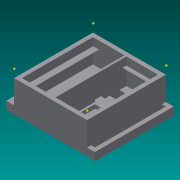
# Autodesk Inventor part: nano_enclosure_v3
Saved by Autodesk Inventor 2015 (Build 190159000, 159)
## iProperties
Created: 2015-03-02
Part Number: nano_enclosure_v3
Material: Generic
Document SubType Name: Modeling
Designer: Jeff
Density: 1 g/cm^3
Appearance: Default
Author: Jeff
Autodesk Inventor part; units mm, degrees
ref_plane "YZ Plane" through (0, 0, 0) normal (1, 0, 0) x (0, 1, 0)
ref_plane "XZ Plane" through (0, 0, 0) normal (0, 1, 0) x (-1, 0, 0)
ref_plane "XY Plane" through (0, 0, 0) normal (0, 0, 1) x (1, 0, 0)
sketch "Sketch2" plane through (0, 0, 0) normal (0, 0, 1) x (1, 0, 0)
  line L0 (0, 0) -> (46.99, 0)
  line L1 (46.99, 0) -> (46.99, 50.8)
  line L2 (46.99, 50.8) -> (0, 50.8)
  line L3 (0, 50.8) -> (0, 0)
  dimension "d0" = 50.8
  dimension "d1" = 46.99
  constraints: 8 end point, 2 parallel, 1 horizontal, 1 perpendicular
  measures "d0" distance of L0.end L1.end
  measures "d1" distance of L1.end L2.end
extrude "Extrusion1" add sketch "Sketch2" along normal blind 25.4
sketch "Sketch3" plane through (0, 0, 25.4) normal (0, 0, 1) x (1, 0, 0)
  line L0 (2.54, 2.54) -> (22.86, 2.54)
  line L1 (22.86, 2.54) -> (22.86, 48.26)
  line L2 (22.86, 48.26) -> (2.54, 48.26)
  line L3 (2.54, 48.26) -> (2.54, 2.54)
  line L4 (0, 0) -> (46.99, 0) projected
  line L5 (0, 50.8) -> (0, 0) projected
  line L6 (46.99, 50.8) -> (0, 50.8) projected
  line L7 (24.13, 2.54) -> (44.45, 2.54)
  line L8 (44.45, 2.54) -> (44.45, 48.26)
  line L9 (44.45, 48.26) -> (24.13, 48.26)
  line L10 (24.13, 48.26) -> (24.13, 2.54)
  line L11 (46.99, 0) -> (46.99, 50.8) projected
  dimension "d4" = 2.54
  dimension "d5" = 2.54
  dimension "d6" = 2.54
  dimension "d7" = 22.86
  dimension "d8" = 2.54
  dimension "d9" = 2.54
  dimension "d10" = 2.54
  dimension "d11" = 22.86
  constraints: 16 end point, 4 parallel, 2 horizontal, 2 perpendicular
  measures "d4" distance between parallel lines of L4 L0
  measures "d5" distance between parallel lines of L5 L3
  measures "d6" distance between parallel lines of L6 L2
  measures "d7" distance between parallel lines of L5 L1
  measures "d8" distance between parallel lines of L4 L7
  measures "d9" distance between parallel lines of L11 L8
  measures "d10" distance between parallel lines of L6 L9
  measures "d11" distance between parallel lines of L11 L10
extrude "Extrusion2" cut sketch "Sketch3" against normal blind 20.32 contours L3 L2 L1 L0 | L10 L9 L8 L7
sketch "Sketch4" plane through (0, 0, 0) normal (0, 0, -1) x (-1, 0, 0)
  circle A0 centre (-12.7, 17.78) radius 8.89
  line L0 (0, 50.8) -> (0, 0) projected
  line L1 (0, 0) -> (-46.99, 0) projected
  dimension "d14" = 17.78
  dimension "d17" = 12.7
  dimension "d18" = 17.78
  constraints: 1 centre point
  measures "d14" diameter of A0
  measures "d17" distance from line of L0 A0.centre
  measures "d18" distance from line of L1 A0.centre
extrude "Extrusion3" cut sketch "Sketch4" against normal blind 3.175
sketch "Sketch5" plane through (0, 0, 0) normal (0, 0, -1) x (-1, 0, 0)
  point P0 (0, 0)
sketch "Sketch6" plane through (12.7, 17.78, 3.175) normal (0, 0, -1) x (-1, 0, 0)
  circle A0 centre (0, 0) radius 8.89 projected
  line L0 (0, 0) -> (-5.08, 0)
  line L1 (-5.08, 0) -> (-5.08, 12.7)
  line L2 (-5.08, 12.7) -> (0, 12.7)
  line L3 (0, 12.7) -> (0, 0)
  line L4 (0, 0) -> (5.08, 0)
  line L5 (5.08, 0) -> (5.08, 12.7)
  line L6 (5.08, 12.7) -> (0, 12.7)
  line L7 (0, 12.7) -> (0, 0)
  point P0 (12.7, -17.78)
  dimension "d21" = 12.7
  dimension "d22" = 5.08
  dimension "d23" = 5.08
  constraints: 16 end point, 4 parallel, 2 horizontal, 2 perpendicular, 1 point on line
  measures "d21" distance between parallel lines of L4 L6
  measures "d22" distance of L0.start L0.end
  measures "d23" distance between parallel lines of L3 L5
extrude "Extrusion4" cut sketch "Sketch6" along normal blind 5.08 contours L5 L4 L3 A0 | A0 L3 L6 L5 | L1 L2 L3 A0 | A0 L3 L0 L1
sketch "Sketch7" plane through (0, 0, 3.175) normal (0, 0, -1) x (-1, 0, 0)
  point P0 (0, 0)
sketch "Sketch8" plane through (0, 0, 3.175) normal (0, 0, -1) x (-1, 0, 0)
  line L0 (-7.62, 25.0756) -> (-7.62, 30.48) projected
  line L1 (-17.78, 30.48) -> (-7.62, 30.48)
  line L2 (-7.62, 30.48) -> (-7.62, 26.67)
  line L3 (-7.62, 26.67) -> (-17.78, 26.67)
  line L4 (-17.78, 26.67) -> (-17.78, 30.48)
  point P0 (0, 0)
  dimension "d26" = 3.81
  constraints: 8 end point, 2 parallel, 1 horizontal, 1 perpendicular, 1 point on line
  measures "d26" distance between parallel lines of L1 L3
extrude "Extrusion5" cut sketch "Sketch8" against normal blind 2.54
sketch "Sketch14" plane through (44.45, 2.54, 25.4) normal (-1, 0, 0) x (0, 0, 1)
  line L0 (0, 0) -> (-20.32, 0) projected
  line L1 (0, 45.72) -> (-20.32, 45.72) projected
  line L2 (-10.16, 45.72) -> (-10.16, 43.18)
  line L3 (-10.16, 43.18) -> (-12.7, 45.72)
  line L4 (-10.16, 0) -> (-10.16, 2.54)
  line L5 (-10.16, 2.54) -> (-12.7, 0)
  point P0 (-25.4, -2.54)
  dimension "d52" = 45
  dimension "d53" = 2.54
  dimension "d54" = 2.54
  dimension "d55" = 45
  dimension "d56" = 7.62
  dimension "d57" = 7.62
  constraints: 8 end point, 2 midpoint, 2 point on line, 1 perpendicular, 1 vertical
  measures "d52" angle of L3 L2
  measures "d53" distance of L2.start L2.end
  measures "d54" distance of L4.start L4.end
  measures "d55" angle of L5 L4
  measures "d56" distance of L0.end L5.end
  measures "d57" distance of L1.end L3.end
extrude "Extrusion11" add sketch "Sketch14" along normal blind 20.32
sketch "Sketch16" plane through (2.54, 2.54, 25.4) normal (0, 1, 0) x (1, 0, 0)
  line L0 (0, 10.16) -> (3.81, 10.16)
  line L1 (3.81, 10.16) -> (0, 13.97)
  line L2 (0, 0) -> (0, 20.32) projected
  line L3 (20.32, 0) -> (20.32, 20.32)
  line L4 (20.32, 13.97) -> (16.51, 10.16)
  line L5 (16.51, 10.16) -> (20.32, 10.16)
  line L6 (20.32, 20.32) -> (0, 20.32) projected
  point P0 (-2.54, 25.4)
  dimension "d60" = 45
  dimension "d61" = 3.81
  dimension "d62" = 3.81
  dimension "d64" = 45
  dimension "d144" = 10.16
  dimension "d145" = 10.16
  constraints: 10 end point, 2 midpoint, 2 point on line, 1 horizontal, 1 parallel
  measures "d60" angle of L4 L5
  measures "d61" distance of L4.end L5.end
  measures "d62" distance of L0.start L0.end
  measures "d64" angle of L1 L0
  measures "d144" distance between parallel lines of L6 L5
  measures "d145" distance between parallel lines of L6 L0
extrude "Extrusion12" add sketch "Sketch16" along normal blind 45.72
sketch "Sketch17" plane through (0, 0, 0) normal (-1, 0, 0) x (0, 0, 1)
  line L0 (0, 50.8) -> (25.4, 50.8) projected
  line L1 (0, 0) -> (5.08, 0)
  line L2 (5.08, 0) -> (5.08, 50.8)
  line L3 (5.08, 50.8) -> (0, 50.8)
  line L4 (0, 50.8) -> (0, 0)
  dimension "d68" = 5.08
  constraints: 8 end point, 2 parallel, 1 horizontal, 1 perpendicular, 1 point on line
  measures "d68" distance between parallel lines of L4 L2
extrude "Extrusion13" add sketch "Sketch17" along normal blind 5.08
sketch "Sketch18" plane through (0, 0, 5.08) normal (0, 0, 1) x (1, 0, 0)
  line L0 (0, 50.8) -> (0, 0) projected
  line L1 (0, 2.54) -> (-2.54, 2.54)
  line L2 (-2.54, 2.54) -> (-2.54, 48.26)
  line L3 (-2.54, 48.26) -> (0, 48.26)
  line L4 (0, 48.26) -> (0, 2.54)
  line L5 (0, 50.8) -> (-5.08, 50.8) projected
  line L6 (0, 0) -> (-5.08, 0) projected
  dimension "d71" = 2.54
  dimension "d72" = 2.54
  dimension "d73" = 2.54
  constraints: 8 end point, 2 parallel, 1 horizontal, 1 perpendicular, 1 point on line
  measures "d71" distance of L2.end L3.end
  measures "d72" distance between parallel lines of L5 L3
  measures "d73" distance between parallel lines of L6 L1
extrude "Extrusion14" cut sketch "Sketch18" against normal blind 5.08
sketch "Sketch19" plane through (46.99, 0, 0) normal (1, 0, 0) x (0, 0, -1)
  line L0 (0, 50.8) -> (-25.4, 50.8) projected
  line L1 (0, 0) -> (-5.08, 0)
  line L2 (-5.08, 0) -> (-5.08, 50.8)
  line L3 (-5.08, 50.8) -> (0, 50.8)
  line L4 (0, 50.8) -> (0, 0)
  dimension "d76" = 5.08
  constraints: 8 end point, 2 parallel, 1 horizontal, 1 perpendicular, 1 point on line
  measures "d76" distance between parallel lines of L4 L2
extrude "Extrusion15" add sketch "Sketch19" along normal blind 5.08
sketch "Sketch21" plane through (46.99, 0, 5.08) normal (0, 0, 1) x (1, 0, 0)
  line L0 (0, 0) -> (0, 50.8) projected
  line L1 (0, 2.54) -> (2.54, 2.54)
  line L2 (2.54, 2.54) -> (2.54, 48.26)
  line L3 (2.54, 48.26) -> (0, 48.26)
  line L4 (0, 48.26) -> (0, 2.54)
  line L5 (0, 50.8) -> (5.08, 50.8) projected
  line L6 (0, 0) -> (5.08, 0) projected
  line L7 (5.08, 50.8) -> (5.08, 0) projected
  point P0 (-46.99, 0)
  dimension "d79" = 2.54
  dimension "d81" = 2.54
  dimension "d82" = 2.54
  constraints: 8 end point, 2 parallel, 1 horizontal, 1 perpendicular, 1 point on line
  measures "d79" distance between parallel lines of L5 L3
  measures "d81" distance between parallel lines of L6 L1
  measures "d82" distance between parallel lines of L7 L2
extrude "Extrusion16" cut sketch "Sketch21" against normal blind 5.08 contours L0 L3 L2 L1
sketch "Sketch23" plane through (0, 0, 5.08) normal (0, 0, 1) x (1, 0, 0)
  line L0 (24.13, 2.54) -> (24.13, 48.26) projected
  line L1 (24.13, 33.02) -> (44.45, 33.02)
  line L2 (44.45, 33.02) -> (44.45, 48.26)
  line L3 (44.45, 48.26) -> (24.13, 48.26)
  line L4 (24.13, 48.26) -> (24.13, 33.02)
  line L5 (24.13, 37.465) -> (31.75, 37.465)
  line L6 (31.75, 37.465) -> (31.75, 43.815)
  line L7 (31.75, 43.815) -> (24.13, 43.815)
  line L8 (24.13, 43.815) -> (24.13, 37.465)
  line L9 (44.45, 48.26) -> (39.37, 48.26)
  line L10 (39.37, 48.26) -> (39.37, 33.02)
  line L11 (39.37, 33.02) -> (44.45, 33.02)
  line L12 (44.45, 33.02) -> (44.45, 48.26)
  point P0 (0, 0)
  dimension "d91" = 15.24
  dimension "d92" = 6.35
  dimension "d93" = 7.62
  dimension "d94" = 4.445
  dimension "d95" = 4.445
  dimension "d96" = 5.08
  constraints: 24 end point, 6 parallel, 3 horizontal, 3 perpendicular, 3 point on line, 1 coincident
  measures "d91" distance between parallel lines of L3 L1
  measures "d92" distance between parallel lines of L7 L5
  measures "d93" distance between parallel lines of L0 L6
  measures "d94" distance between parallel lines of L1 L5
  measures "d95" distance between parallel lines of L3 L7
  measures "d96" distance between parallel lines of L2 L10
extrude "Extrusion21" cut sketch "Sketch23" against normal blind 25.4 contours L0 L7 L6 L5
extrude "Extrusion22" cut sketch "Sketch23" against normal blind 1.27 contours L0 L5 L6 L7 L3 L10 L1
extrude "Extrusion23" cut sketch "Sketch23" against normal blind 2.54 contours L10 L3 L2 L1
sketch "Sketch27" plane through (24.13, 2.54, 25.4) normal (1, 0, 0) x (0, 0, -1)
  line L0 (20.32, 0) -> (20.32, 30.48) projected
  line L1 (20.32, 10.16) -> (19.05, 10.16)
  line L2 (19.05, 10.16) -> (19.05, 15.24)
  line L3 (19.05, 15.24) -> (20.32, 15.24)
  line L4 (20.32, 15.24) -> (20.32, 10.16)
  line L5 (20.32, 25.4) -> (19.05, 25.4)
  line L6 (19.05, 25.4) -> (19.05, 30.48)
  line L7 (19.05, 30.48) -> (20.32, 30.48)
  line L8 (20.32, 30.48) -> (20.32, 25.4)
  line L9 (12.7, 0) -> (20.32, 0) projected
  line L10 (12.7, 45.72) -> (21.59, 45.72) projected
  point P0 (25.4, -2.54)
  dimension "d133" = 1.27
  dimension "d134" = 5.08
  dimension "d135" = 5.08
  dimension "d136" = 10.16
  dimension "d137" = 10.16
  dimension "d138" = 15.24
  constraints: 16 end point, 4 parallel, 2 horizontal, 2 perpendicular, 2 point on line, 1 vertical alignment
  measures "d133" distance between parallel lines of L0 L2
  measures "d134" distance between parallel lines of L3 L1
  measures "d135" distance between parallel lines of L7 L5
  measures "d136" distance between parallel lines of L5 L3
  measures "d137" distance between parallel lines of L9 L1
  measures "d138" distance between parallel lines of L10 L7
extrude "Extrusion25" cut sketch "Sketch27" against normal blind 2.54
sketch "Sketch28" plane through (0, 0, 25.4) normal (-1, 0, 0) x (0, 0, 1)
  line L0 (-20.32, 0) -> (0, 0) projected
  line L1 (0, 50.8) -> (-5.08, 50.8)
  line L2 (-5.08, 50.8) -> (-5.08, 0)
  line L3 (-5.08, 0) -> (0, 0)
  line L4 (0, 0) -> (0, 50.8)
  point P0 (-25.4, 0)
  dimension "d141" = 5.08
  constraints: 8 end point, 2 parallel, 1 horizontal, 1 perpendicular, 1 point on line
  measures "d141" distance between parallel lines of L2 L4
extrude "Extrusion26" cut sketch "Sketch28" against normal blind 50.8
sketch "Sketch29" plane through (0, 0, 5.08) normal (0, 0, 1) x (1, 0, 0)
  point P0 (0, 0)
sketch "Sketch30" plane through (0, 0, 5.08) normal (0, 0, 1) x (1, 0, 0)
  line L0 (25.4, 6.35) -> (43.18, 6.35)
  line L1 (43.18, 6.35) -> (43.18, 26.67)
  line L2 (43.18, 26.67) -> (25.4, 26.67)
  line L3 (25.4, 26.67) -> (25.4, 6.35)
  line L4 (24.13, 2.54) -> (24.13, 12.7) projected
  line L5 (44.45, 33.02) -> (44.45, 2.54) projected
  line L6 (44.45, 2.54) -> (24.13, 2.54) projected
  point P0 (0, 0)
  dimension "d146" = 1.27
  dimension "d147" = 1.27
  dimension "d148" = 20.32
  dimension "d149" = 3.81
  dimension "d150" = 17.78
  constraints: 8 end point, 2 parallel, 1 horizontal, 1 perpendicular
  measures "d146" distance between parallel lines of L4 L3
  measures "d147" distance between parallel lines of L5 L1
  measures "d148" distance between parallel lines of L2 L0
  measures "d149" distance between parallel lines of L6 L0
  measures "d150" distance between parallel lines of L3 L1
extrude "Extrusion27" cut sketch "Sketch30" against normal blind 2.54
body "Solid1"
